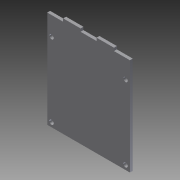
# Autodesk Inventor part: board uvtron
Saved by Autodesk Inventor 2012 (Build 160160000, 160)
## iProperties
Created: 2013-12-07
Part Number: board uvtron
Material: Default
Document SubType Name: Modeling
Designer: Irwan Haryanto
Density: 1 g/cm^3
Author: Irwan Haryanto
Autodesk Inventor part; units mm, degrees
ref_plane "YZ Plane" through (0, 0, 0) normal (1, 0, 0) x (0, 1, 0)
ref_plane "XZ Plane" through (0, 0, 0) normal (0, 1, 0) x (-1, 0, 0)
ref_plane "XY Plane" through (0, 0, 0) normal (0, 0, 1) x (1, 0, 0)
sketch "Sketch1" plane through (0, 0, 0) normal (0, 0, 1) x (1, 0, 0)
  line L0 (25.99, 41.9307) -> (25.99, -25.0693)
  line L1 (25.99, -25.0693) -> (-31.01, -25.0693)
  line L2 (-31.01, -25.0693) -> (-31.01, 41.9307)
  circle A0 centre (-28.01, -22.0693) radius 1.5
  circle A1 centre (22.99, -22.0693) radius 1.5
  circle A2 centre (-28.01, 28.9307) radius 1.5
  circle A3 centre (22.99, 28.9307) radius 1.5
  line L3 (-20.01, 41.9307) -> (-20.01, 43.9307)
  line L4 (-20.01, 43.9307) -> (-8.01, 43.9307)
  line L5 (-8.01, 43.9307) -> (-8.01, 41.9307)
  line L6 (2.99, 41.9307) -> (2.99, 43.9307)
  line L7 (2.99, 43.9307) -> (14.99, 43.9307)
  line L8 (14.99, 43.9307) -> (14.99, 41.9307)
  line L9 (-31.01, 41.9307) -> (-20.01, 41.9307)
  line L10 (-8.01, 41.9307) -> (2.99, 41.9307)
  line L11 (14.99, 41.9307) -> (25.99, 41.9307)
  point P0 (0, 0)
  dimension "d0" = 57
  dimension "d1" = 67
  dimension "d2" = 3
  dimension "d3" = 3
  dimension "d4" = 3
  dimension "d5" = 51
  dimension "d6" = 51
  dimension "d7" = 51
  dimension "d8" = 51
  dimension "d9" = 3
  dimension "d10" = 2
  dimension "d11" = 12
  dimension "d12" = 12
  dimension "d13" = 11
  dimension "d14" = 11
  dimension "d15" = 3
  dimension "d16" = 3
  dimension "d17" = 3
  constraints: 24 end point, 11 perpendicular, 6 parallel, 4 centre point, 3 horizontal
  measures "d0" distance of L0.end L2.start
  measures "d1" distance of L0.start L0.end
  measures "d2" diameter of A1
  measures "d3" diameter of A0
  measures "d4" diameter of A2
  measures "d5" distance of A1.centre A0.centre
  measures "d6" distance of A0.centre A2.centre
  measures "d7" distance of A2.centre A3.centre
  measures "d8" distance of A1.centre A3.centre
  measures "d9" distance from line of L2 A0.centre
  measures "d10" distance of L9.end L3.end
  measures "d11" distance of L3.end L4.end
  measures "d12" distance of L6.end L7.end
  measures "d13" distance between parallel lines of L3 L2
  measures "d14" distance between parallel lines of L6 L5
  measures "d15" distance from line of L1 A0.centre
  measures "d16" distance from line of L1 A1.centre
  measures "d17" distance from line of L2 A2.centre
extrude "Extrusion1" add sketch "Sketch1" along normal blind 2 contours L0 L1 L2 L9 L3 L4 L5 L10 L6 L7 L8 L11 | A0 | A1 | A2 | A3
sketch "Sketch2" plane through (0, 0, 2) normal (0, 0, 1) x (1, 0, 0)
  line L0 (-31.01, -25.0693) -> (-31.01, 41.9307)
  line L1 (25.99, 41.9307) -> (25.99, -25.0693)
  circle A0 centre (22.99, 28.9307) radius 1.5
  line L2 (-31.01, 41.9307) -> (-20.01, 41.9307)
  line L3 (-8.01, 41.9307) -> (2.99, 41.9307)
  line L4 (-20.01, 41.9307) -> (-20.01, 43.9307)
  line L5 (-20.01, 43.9307) -> (-8.01, 43.9307)
  line L6 (-8.01, 43.9307) -> (-8.01, 41.9307)
  line L7 (14.99, 41.9307) -> (25.99, 41.9307)
  line L8 (2.99, 41.9307) -> (2.99, 43.9307)
  line L9 (2.99, 43.9307) -> (14.99, 43.9307)
  line L10 (14.99, 43.9307) -> (14.99, 41.9307)
  circle A1 centre (-28.01, -22.0693) radius 1.5
  circle A2 centre (22.99, -22.0693) radius 1.5
  line L11 (25.99, -25.0693) -> (-31.01, -25.0693)
  circle A3 centre (-28.01, 28.9307) radius 1.5
  point P0 (0, 0)
  point P1 (0, 0)
  dimension "d20" = 57
  dimension "d21" = 67
  dimension "d22" = 3
  dimension "d23" = 3
  dimension "d24" = 3
  dimension "d25" = 51
  dimension "d26" = 51
  dimension "d27" = 51
  dimension "d28" = 51
  dimension "d29" = 3
  dimension "d30" = 2
  dimension "d31" = 12
  dimension "d32" = 12
  dimension "d33" = 11
  dimension "d34" = 11
  dimension "d35" = 3
  dimension "d36" = 3
  dimension "d37" = 3
  constraints: 24 end point, 11 perpendicular, 6 parallel, 4 centre point, 3 horizontal
  measures "d20" distance of L11.start L0.start
  measures "d21" distance of L7.end L11.start
  measures "d22" diameter of A2
  measures "d23" diameter of A1
  measures "d24" diameter of A3
  measures "d25" distance of A2.centre A1.centre
  measures "d26" distance of A1.centre A3.centre
  measures "d27" distance of A3.centre A0.centre
  measures "d28" distance of A2.centre A0.centre
  measures "d29" distance from line of L0 A1.centre
  measures "d30" distance of L4.start L4.end
  measures "d31" distance of L4.end L6.start
  measures "d32" distance of L9.start L9.end
  measures "d33" distance between parallel lines of L4 L0
  measures "d34" distance between parallel lines of L8 L6
  measures "d35" distance from line of L11 A1.centre
  measures "d36" distance from line of L11 A2.centre
  measures "d37" distance from line of L0 A3.centre
hole "Hole1" at (-28.01, 28.9307, 2) at (22.99, 28.9307, 2) at (22.99, -22.0693, 2) at (-28.01, -22.0693, 2) direction (0, 0, -1) diameter 3 end through all
body "Solid1"
